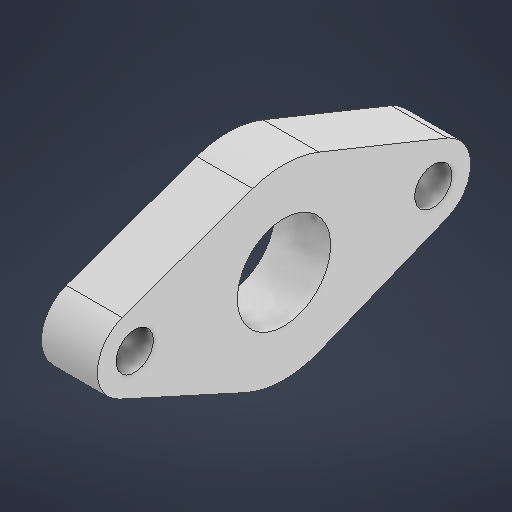
# Autodesk Inventor part: Part5
Saved by Autodesk Inventor 2026 (Build 300175050, 175E)
## iProperties
Created: 2026-03-26
Part Number: Part5
Material: Generic
Document SubType Name: Modeling
Designer: Administrator
Density: 1 g/cm^3
Appearance: Default
Author: Administrator
Autodesk Inventor part; units mm, degrees
ref_plane "YZ Plane" through (0, 0, 0) normal (1, 0, 0) x (0, 1, 0)
ref_plane "XZ Plane" through (0, 0, 0) normal (0, 1, 0) x (-1, 0, 0)
ref_plane "XY Plane" through (0, 0, 0) normal (0, 0, 1) x (1, 0, 0)
sketch "Sketch1" plane through (0, 0, 0) normal (1, 0, 0) x (0, 1, 0)
  circle A0 centre (0, 0) radius 12.5
  circle A1 centre (0, -40) radius 5
  circle A2 centre (1.7099, 39.9817) radius 5
  arc A3 (11.1326, 43.3305) -> (-7.3924, 44.1227) centre (1.7099, 39.9817) ccw
  arc A4 (-9.2702, -43.75) -> (9.2702, -43.75) centre (0, -40) ccw
  line L0 (11.1326, 43.3305) -> (23.5566, 8.3718)
  line L1 (-7.3924, 44.1227) -> (-22.7558, 10.3525)
  line L2 (9.2702, -43.75) -> (23.1756, -9.375)
  line L3 (-9.2702, -43.75) -> (-23.1756, -9.375)
  arc A5 (23.1756, -9.375) -> (23.5566, 8.3718) centre (0, 0) ccw
  arc A6 (-22.7558, 10.3525) -> (-23.1756, -9.375) centre (0, 0) ccw
  line L4 (0, 40.7596) -> (0, -40)
  dimension "d0" = 40
  dimension "d1" = 80
  dimension "d2" = 10
  dimension "d3" = 25
  dimension "d4" = 10
  dimension "d6" = 20
  dimension "d7" = 20
  constraints: 10 end point, 8 point on circle, 8 tangent, 7 centre point, 4 coincident, 1 vertical
  measures "d0" distance of A1.centre point (0, 0)
  measures "d1" distance of A1.centre A2.centre
  measures "d2" diameter of A2
  measures "d3" diameter of A0
  measures "d4" diameter of A1
  measures "d6" diameter of A3
  measures "d7" diameter of A4
extrude "Extrusion1" add sketch "Sketch1" along normal mid plane 15
body "Solid1"
